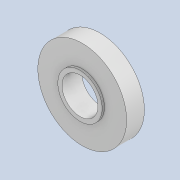
# Autodesk Inventor part: 1ギア補強材
Saved by Autodesk Inventor 2020.4 (Build 244396000, 396)
## iProperties
Created: 2021-04-23
Part Number: 1ギア補強材
Material: アルミニウム 2014-T4
Document SubType Name: Modeling
Designer: happy
Density: 2.8 g/cm^3
Appearance: サテン
Author: happy
Autodesk Inventor part; units mm, degrees
ref_plane "YZ Plane" through (0, 0, 0) normal (1, 0, 0) x (0, 1, 0)
ref_plane "XZ Plane" through (0, 0, 0) normal (0, 1, 0) x (-1, 0, 0)
ref_plane "XY Plane" through (0, 0, 0) normal (0, 0, 1) x (1, 0, 0)
sketch "スケッチ1" plane through (0, 0, 0) normal (0, 0, 1) x (1, 0, 0)
  circle A0 centre (0, 0) radius 5
  circle A1 centre (0, 0) radius 2.025
  dimension "d0" = 10
  dimension "d1" = 4.05
  constraints: 2 centre point, 2 coincident
  measures "d0" diameter of A0
  measures "d1" diameter of A1
extrude "押し出し1" add sketch "スケッチ1" along normal blind 2
sketch "スケッチ2" plane through (0, 0, 2) normal (0, 0, 1) x (1, 0, 0)
  circle A0 centre (0, 0) radius 5 projected
  circle A1 centre (0, 0) radius 2.025 projected
  circle A2 centre (0, 0) radius 2.5
  dimension "d4" = 5
  constraints: 1 centre point, 1 coincident
  measures "d4" diameter of A2
extrude "押し出し2" add sketch "スケッチ2" along normal blind 0.25 contours A2
